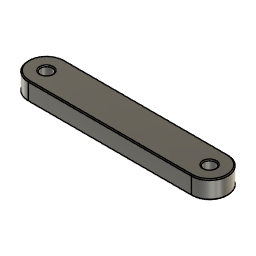
Coupler v4 (Autodesk Fusion 360 design; units mm, degrees)
Autodesk Fusion 360 part; units mm, degrees
sketch "Sketch1" plane through (0, 0, 0) normal (0, 0, 1) x (1, 0, 0)
  circle A0 centre (0, 0) radius 3.275
  circle A1 centre (0, 0) radius 10
  line L0 (0, 0) -> (90, 0) construction
  circle A2 centre (90, 0) radius 3.275
  circle A3 centre (90, 0) radius 10
  line L1 (0, 10) -> (90, 10)
  line L2 (0, -10) -> (90, -10)
  dimension "d1" = 6.55
  dimension "d2" = 20
  dimension "d4" = 90
  dimension "d5" = 6.55
  dimension "d6" = 20
  constraint coincident A0.centre A1.centre
  constraint horizontal L0
  constraint coincident L0.end A2.centre
  constraint concentric A2 A3
  constraint coincident A1 L1.start
  constraint coincident A3 L1.end
  constraint tangent A3 L1
  constraint coincident A1 L2.start
  constraint coincident A3 L2.end
  constraint tangent A3 L2
  constraint tangent A1 L1
  constraint tangent A1 L2
  measures "d1" diameter of A0
  measures "d2" diameter of A1
  measures "d4" distance of A0.centre L0.end
  measures "d5" diameter of A2
  measures "d6" diameter of A3
extrude "Extrude1" add sketch "Sketch1" along normal blind 10
chamfer "Chamfer1" distance 0.5 angle 45 2 faces at (59.0164, 7.1403, 0) (59.0164, 7.1403, 10)
equation "length = 90 mm"
equation "d4 = length"
